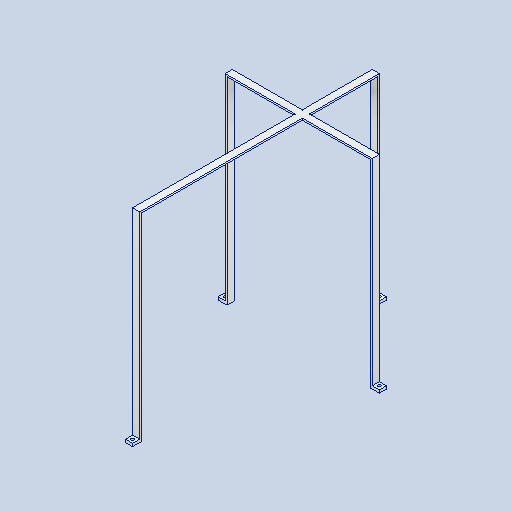
# Autodesk Inventor part: Soporte
Saved by Autodesk Inventor 2022.1 (Build 261234000, 234)
## iProperties
Created: 2021-10-03
Part Number: Soporte
Material: Aluminio 6061
Document SubType Name: Sheet Metal
Designer: seb_0
Density: 2.7 g/cm^3
Appearance: Aluminio - Plano
Flat Pattern Width: 35.52 cm
Flat Pattern Length: 27.936 cm
Flat Pattern Area: 992.287 cm^2
Sheet Metal Rule: Por defecto
Sheet Metal Width: 355.200 mm
Sheet Metal Length: 279.360 mm
Sheet Metal Area: 99228.672 mm^2
Author: seb_0
Autodesk Inventor part; units mm, degrees
ref_plane "YZ Plane" through (0, 0, 0) normal (1, 0, 0) x (0, 1, 0)
ref_plane "XZ Plane" through (0, 0, 0) normal (0, 1, 0) x (-1, 0, 0)
ref_plane "XY Plane" through (0, 0, 0) normal (0, 0, 1) x (1, 0, 0)
sketch "Boceto1" plane through (0, 0, 0) normal (0, 1, 0) x (-1, 0, 0)
  line L0 (0, 5) -> (0, -5)
  line L1 (200.66, -5) -> (200.66, 5)
  line L2 (105.33, 229.87) -> (95.33, 229.87)
  line L3 (95.33, 229.87) -> (95.33, -100.33)
  line L4 (95.33, -100.33) -> (105.33, -100.33)
  line L5 (105.33, -100.33) -> (105.33, 229.87)
  line L6 (200.66, 0) -> (0, 0)
  circle A0 centre (162.56, 102.87) radius 10 projected
  circle A1 centre (38.1, 102.87) radius 10 projected
  line L7 (200.66, 77.47) -> (200.66, 217.17) projected
  line L8 (187.96, 229.87) -> (12.7, 229.87) projected
  line L9 (0, 217.17) -> (0, 77.47) projected
  line L10 (12.7, 64.77) -> (187.96, 64.77) projected
  line L11 (200.66, 5) -> (105.33, 229.87)
  line L12 (95.33, 229.87) -> (0, 5)
  circle A2 centre (162.56, -62.23) radius 10 projected
  circle A3 centre (38.1, -62.23) radius 10 projected
  line L13 (200.66, -87.63) -> (200.66, 52.07) projected
  line L14 (187.96, 64.77) -> (12.7, 64.77) projected
  line L15 (0, 52.07) -> (0, -87.63) projected
  line L16 (12.7, -100.33) -> (187.96, -100.33) projected
  line L17 (0, -5) -> (200.66, -5)
  line L18 (200.66, 5) -> (0, 5)
  arc A4 (187.96, -100.33) -> (200.66, -87.63) centre (187.96, -87.63) ccw projected
  arc A5 (200.66, 52.07) -> (187.96, 64.77) centre (187.96, 52.07) ccw projected
  arc A6 (12.7, 64.77) -> (0, 52.07) centre (12.7, 52.07) ccw projected
  arc A7 (0, -87.63) -> (12.7, -100.33) centre (12.7, -87.63) ccw projected
  arc A8 (187.96, 64.77) -> (200.66, 77.47) centre (187.96, 77.47) ccw projected
  arc A9 (200.66, 217.17) -> (187.96, 229.87) centre (187.96, 217.17) ccw projected
  arc A10 (12.7, 229.87) -> (0, 217.17) centre (12.7, 217.17) ccw projected
  arc A11 (0, 77.47) -> (12.7, 64.77) centre (12.7, 77.47) ccw projected
  point P0 (0, 0)
  point P1 (100.33, -100.33)
  point P2 (105.33, 5)
  point P3 (105.33, 0)
  point P4 (95.33, 5)
  point P5 (95.33, -5)
  point P6 (105.33, -5)
  dimension "d2" = 10
  constraints: 22 end point, 4 midpoint, 3 parallel, 2 equal length, 2 horizontal, 2 perpendicular, 1 coincident, 1 point on line
  measures "d2" distance of L1.start L1.end
extrude "Extrusión1" add sketch "Boceto1" along normal blind 2.5 contours L18 L3 L6 L0 | L6 L3 L17 L0 | L18 L5 L6 L3 | L3 L10 L5 L18 | L6 L5 L17 L3 | L3 L2 L5 L10 | L18 L1 L6 L5 | L17 L5 L4 L3 | L6 L1 L17 L5
sketch "Boceto2" plane through (-105.33, 0, 229.87) normal (0, 0, 1) x (1, 0, 0)
  line L0 (0, 0) -> (10, 0) projected
  line L1 (10, 0) -> (10, 2.5) projected
  line L2 (0, 2.5) -> (10, 2.5) projected
  line L3 (0, 0) -> (0, 2.5) projected
  line L4 (0, 0) -> (0, 2.5) projected
  line L5 (0, 0) -> (0, -276.86)
  line L6 (0, -276.86) -> (10, -276.86)
  line L7 (0, 0) -> (10, 0) projected
  line L8 (10, -276.86) -> (10, 0)
  line L9 (92.63, -276.86) -> (-82.63, -276.86) projected
  line L10 (92.63, 0) -> (-82.63, 0) projected
  line L11 (-82.63, 0) -> (-82.63, -276.86) projected
  line L12 (92.63, -276.86) -> (92.63, 0) projected
  point P0 (5, -276.86)
  constraints: 6 end point, 2 midpoint, 2 perpendicular, 1 vertical
extrude "Extrusión2" add sketch "Boceto2" along normal blind 2.5 contours L3 L2 L1 L0 | L0 L8 L6 L5
sketch "Boceto3" plane through (-95.33, 0, -100.33) normal (0, 0, -1) x (-1, 0, 0)
  line L0 (0, 0) -> (10, 0) projected
  line L1 (10, 0) -> (10, 2.5) projected
  line L2 (0, 2.5) -> (10, 2.5) projected
  line L3 (0, 0) -> (0, 2.5) projected
  line L4 (10, 0) -> (0, 0) projected
  line L5 (0, -276.86) -> (0, 0) projected
  line L6 (10, -276.86) -> (0, -276.86) projected
  line L7 (10, 0) -> (10, -276.86) projected
  point P0 (-95.33, 0)
extrude "Extrusión3" add sketch "Boceto3" along normal blind 2.5
sketch "Boceto4" plane through (0, 0, 5) normal (1, 0, 0) x (0, 0, -1)
  line L0 (0, 0) -> (10, 0) projected
  line L1 (10, 0) -> (10, 2.5) projected
  line L2 (0, 2.5) -> (10, 2.5) projected
  line L3 (0, 0) -> (0, 2.5) projected
  line L4 (0, 0) -> (0, -276.86)
  line L5 (0, -276.86) -> (10, -276.86)
  line L6 (10, -276.86) -> (10, 0)
  line L7 (105.33, 0) -> (105.33, -276.86) projected
  point P0 (5, 0)
  constraints: 6 end point, 2 perpendicular, 1 parallel, 1 vertical
extrude "Extrusión4" add sketch "Boceto4" along normal blind 2.5
sketch "Boceto5" plane through (-200.66, 0, -5) normal (-1, 0, 0) x (0, 0, 1)
  line L0 (0, 0) -> (10, 0) projected
  line L1 (10, 0) -> (10, 2.5) projected
  line L2 (0, 2.5) -> (10, 2.5) projected
  line L3 (10, 0) -> (0, 0) projected
  line L4 (0, -276.86) -> (0, 0) projected
  line L5 (10, -276.86) -> (0, -276.86) projected
  line L6 (10, 0) -> (10, -276.86) projected
  line L7 (0, 0) -> (0, 2.5) projected
  point P0 (5, 0)
extrude "Extrusión5" add sketch "Boceto5" along normal blind 2.5
sketch "Boceto6" plane through (-200.66, -276.86, -5) normal (0, -1, 0) x (1, 0, 0)
  line L0 (200.66, 10) -> (200.66, 0) projected
  line L1 (200.66, 0) -> (203.16, 0) projected
  line L2 (203.16, 10) -> (203.16, 0) projected
  line L3 (200.66, 10) -> (203.16, 10) projected
  line L4 (95.33, 234.87) -> (105.33, 234.87) projected
  line L5 (105.33, 234.87) -> (105.33, 237.37) projected
  line L6 (95.33, 237.37) -> (105.33, 237.37) projected
  line L7 (95.33, 234.87) -> (95.33, 237.37) projected
  line L8 (0, 0) -> (0, 10) projected
  line L9 (0, 10) -> (-2.5, 10) projected
  line L10 (-2.5, 0) -> (-2.5, 10) projected
  line L11 (0, 0) -> (-2.5, 0) projected
  line L12 (105.33, -95.33) -> (95.33, -95.33) projected
  line L13 (95.33, -95.33) -> (95.33, -97.83) projected
  line L14 (105.33, -97.83) -> (95.33, -97.83) projected
  line L15 (105.33, -95.33) -> (105.33, -97.83) projected
  line L16 (105.33, -97.83) -> (105.33, -107.83)
  line L17 (105.33, -107.83) -> (95.33, -107.83)
  line L18 (95.33, -97.83) -> (105.33, -97.83) projected
  line L19 (95.33, -107.83) -> (95.33, -97.83)
  line L20 (203.16, 0) -> (213.16, 0)
  line L21 (213.16, 0) -> (213.16, 10)
  line L22 (213.16, 10) -> (203.16, 10)
  line L23 (95.33, 10) -> (95.33, 237.37) projected
  line L24 (95.33, 237.37) -> (95.33, 247.37)
  line L25 (95.33, 247.37) -> (105.33, 247.37)
  line L26 (105.33, 247.37) -> (105.33, 237.37)
  line L27 (-2.5, 0) -> (-2.5, 10) projected
  line L28 (-2.5, 0) -> (-12.5, 0)
  line L29 (-12.5, 0) -> (-12.5, 10)
  line L30 (-12.5, 10) -> (-2.5, 10)
  circle A0 centre (-7.5, 5) radius 2.1
  circle A1 centre (100.33, 242.37) radius 2.1
  circle A2 centre (100.33, -102.83) radius 2.1
  circle A3 centre (208.16, 5) radius 2.1
  point P0 (200.66, 5)
  point P1 (-7.5, 10)
  point P2 (100.33, -107.83)
  dimension "d16" = 4.2
  dimension "d17" = 5
  dimension "d18" = 5
  dimension "d19" = 4.2
  dimension "d20" = 5
  dimension "d21" = 5
  dimension "d22" = 4.2
  dimension "d23" = 5
  dimension "d24" = 5
  dimension "d25" = 4.2
  dimension "d26" = 5
  dimension "d27" = 5
  constraints: 24 end point, 11 perpendicular, 4 centre point, 2 horizontal, 2 midpoint, 2 vertical, 1 parallel
  measures "d16" diameter of A0
  measures "d17" distance of point (-7.5, 10) A0.centre
  measures "d18" distance from line of L10 A0.centre
  measures "d19" diameter of A1
  measures "d20" distance from line of L24 A1.centre
  measures "d21" distance from line of L6 A1.centre
  measures "d22" diameter of A2
  measures "d23" distance of point (100.33, -107.83) A2.centre
  measures "d24" distance from line of L16 A2.centre
  measures "d25" diameter of A3
  measures "d26" distance from line of L22 A3.centre
  measures "d27" distance from line of L2 A3.centre
extrude "Extrusión6" add sketch "Boceto6" against normal blind 4 contours L22 L21 L20 L2 | L24 L25 L26 L6 | L28 L29 L30 L10 | L16 L17 L19 L14
equation "\"d16\" = d19"
equation "\"d22\" = d19"
equation "\"d25\" = d19"
equation "\"Radio_pliegue\" = Grosor"
equation "\"Anchura_desahogo_plegado\" = Grosor"
equation "\"Profundidad_desahogo_plegado\" = 0.5 * Grosor"
equation "\"Tamaño_destalonado\" = 4 * Grosor"
equation "\"Remanente_mínimo\" = 2 * Grosor"
equation "\"Radiodetransición\" = Radio_pliegue"
equation "\"Tamaño_de_radio_de_Jacobi\" = Radio_pliegue"
equation "\"TamañoSeparación\" = Grosor"
equation "\"Grosor\" = 3.048"
